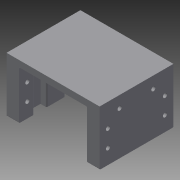
# Autodesk Inventor part: BaseMount
Saved by Autodesk Inventor 2015 (Build 190159000, 159)
## iProperties
Created: 2016-12-14
Part Number: BaseMount
Material: Generic
Document SubType Name: Modeling
Designer: Rudge-Top
Density: 1 g/cm^3
Appearance: Default
Author: Rudge-Top
Autodesk Inventor part; units mm, degrees
ref_plane "YZ Plane" through (0, 0, 0) normal (1, 0, 0) x (0, 1, 0)
ref_plane "XZ Plane" through (0, 0, 0) normal (0, 1, 0) x (-1, 0, 0)
ref_plane "XY Plane" through (0, 0, 0) normal (0, 0, 1) x (1, 0, 0)
sketch "Sketch1" plane through (0, 0, 0) normal (1, 0, 0) x (0, 1, 0)
  line L0 (0, 0) -> (-35, 0)
  line L1 (-35, 0) -> (-35, -23)
  line L2 (-35, -23) -> (0, -23)
  line L3 (0, -23) -> (0, 0)
  dimension "d0" = 35
  dimension "d1" = 23
  constraints: 8 end point, 2 parallel, 1 horizontal, 1 perpendicular
  measures "d0" distance of L2.end L1.end
  measures "d1" distance of L1.end L0.end
extrude "Extrusion1" add sketch "Sketch1" along normal blind 3
sketch "Sketch2" plane through (3, 0, 0) normal (1, 0, 0) x (0, 0, -1)
  line L0 (0, 0) -> (-3, 0)
  line L1 (-3, 0) -> (-3, -35)
  line L2 (-3, -35) -> (0, -35)
  line L3 (0, -35) -> (0, 0)
  dimension "d4" = 3
  dimension "d5" = 35
  constraints: 8 end point, 2 parallel, 1 horizontal, 1 perpendicular
  measures "d4" distance of L2.end L1.end
  measures "d5" distance of L1.end L0.end
extrude "Extrusion2" add sketch "Sketch2" against normal blind 44.1
sketch "Sketch3" plane through (0, -35, 0) normal (0, 0, -1) x (-1, 0, 0)
  line L0 (41.1, 0) -> (38.1, 0)
  line L1 (38.1, 0) -> (38.1, 35)
  line L2 (38.1, 35) -> (41.1, 35)
  line L3 (41.1, 35) -> (41.1, 0)
  point P0 (0, 35)
  dimension "d11" = 21
  dimension "d12" = 4.9
  dimension "d13" = 7
  dimension "d8" = 3
  constraints: 8 end point, 2 parallel, 1 horizontal, 1 perpendicular
  measures "d8" distance of L1.end L2.end
extrude "Extrusion3" add sketch "Sketch3" along normal blind 23
sketch "Sketch4" plane through (0, 0, 0) normal (-1, 0, 0) x (0, 0, 1)
  line L0 (0, 0) -> (0, -35) projected
  line L1 (-23, 0) -> (0, 0) projected
  line L2 (-23, -35) -> (-23, 0) projected
  line L3 (0, -35) -> (-23, -35) projected
  line L4 (0, -28) -> (-23, -28)
  line L5 (-23, -28) -> (-23, -7)
  line L6 (-23, -7) -> (0, -7)
  line L7 (0, -7) -> (0, -28)
  line L8 (-4.9, -28) -> (-4.9, -7)
  dimension "d11" = 21
  dimension "d12" = 4.9
  dimension "d13" = 7
  constraints: 10 end point, 4 point on line, 2 parallel, 2 perpendicular, 1 horizontal
  measures "d11" distance of L4.end L5.end
  measures "d12" distance between parallel lines of L0 L8
  measures "d13" distance between parallel lines of L3 L4
extrude "Extrusion4" add sketch "Sketch4" along normal blind 2.9 contours L0 L6 L2 L1 | L0 L4 L8 L6 | L0 L3 L2 L4
sketch "Sketch5" plane through (-38.1, -35, 0) normal (1, 0, 0) x (0, 0, -1)
  line L0 (0, 0) -> (0, 35) projected
  line L1 (0, 0) -> (23, 0) projected
  line L2 (23, 35) -> (23, 0) projected
  line L3 (0, 35) -> (23, 35) projected
  line L4 (0, 17.5) -> (23, 17.5)
  line L5 (5.9, 21.9028) -> (23, 21.9028)
  line L6 (23, 21.9028) -> (23, 27.9028)
  line L7 (23, 27.9028) -> (5.9, 27.9028)
  line L8 (5.9, 27.9028) -> (5.9, 21.9028)
  line L9 (23, 0) -> (23, 35)
  line L10 (5.9, 13.0972) -> (23, 13.0972)
  line L11 (23, 7.0972) -> (5.9, 7.0972)
  line L12 (5.9, 7.0972) -> (5.9, 13.0972)
  line L13 (23, 13.0972) -> (23, 7.0972)
  line L14 (23, 35) -> (23, 0) projected
  dimension "d16" = 6
  dimension "d17" = 0
  dimension "d18" = 5.9
  constraints: 20 end point, 6 symmetric about line, 2 midpoint, 2 parallel, 1 collinear, 1 horizontal, 1 perpendicular
  measures "d16" distance of L6.end L5.end
  measures "d17" distance between parallel lines of L2 L6
  measures "d18" distance between parallel lines of L0 L8
extrude "Extrusion5" add sketch "Sketch5" along normal blind 2.9 contours L0 L4 L2 L10 L12 L11 L1 | L0 L3 L2 L7 L8 L5 L4
fillet "Fillet1" radius 0.5 2 edges at (-2.9, -17.5, 0) (-35.2, -17.5, 0)
fillet "Fillet2" radius 0.5 6 edges at (-1.45, -7, -4.9) (-1.45, -28, -4.9) (-36.65, -7.0972, -5.9) (-36.65, -13.0972, -5.9) (-36.65, -21.9028, -5.9) (-35.2, -27.9028, -14.45)
sketch "Sketch6" plane through (3, 0, 0) normal (1, 0, 0) x (0, 0, -1)
  line L0 (-3, -35) -> (23, -35) projected
  line L1 (23, -35) -> (23, 0) projected
  line L2 (23, 0) -> (-3, 0) projected
  line L3 (-3, 0) -> (-3, -35) projected
  line L4 (23, -28) -> (23, -7) projected
  line L5 (23, -17.5) -> (9.3491, -17.5)
  line L6 (5.9, -28.4028) -> (23, -28.4028) projected
  line L7 (5.9, -28.4028) -> (5.9, -22.4028) projected
  arc A0 (6.4, -21.9028) -> (5.9, -22.4028) centre (6.4, -22.4028) ccw projected
  line L8 (6.4, -21.9028) -> (23, -21.9028) projected
  line L9 (23, -21.9028) -> (23, -13.0972) projected
  line L10 (23, -13.0972) -> (6.4, -13.0972) projected
  arc A1 (5.9, -12.5972) -> (6.4, -13.0972) centre (6.4, -12.5972) ccw projected
  line L11 (5.9, -12.5972) -> (5.9, -7.5972) projected
  arc A2 (6.4, -7.0972) -> (5.9, -7.5972) centre (6.4, -7.5972) ccw projected
  line L12 (6.4, -7.0972) -> (23, -7.0972) projected
  line L13 (23, -7.0972) -> (23, 0) projected
  line L14 (23, 0) -> (0.5, 0) projected
  line L15 (0.5, -35) -> (0.5, 0) projected
  line L16 (0.5, -35) -> (23, -35) projected
  line L17 (23, -35) -> (23, -28.4028) projected
  line L18 (0, -35) -> (0.5, -35) projected
  line L19 (0.5, -35) -> (0.5, 0) projected
  line L20 (0.5, 0) -> (0, 0) projected
  line L21 (0, 0) -> (0, -35) projected
  point P0 (2.5, -25.5)
  point P1 (16, -31)
  point P2 (8, -31)
  point P3 (2.5, -9.5)
  point P4 (16, -4)
  point P5 (8, -4)
  dimension "d23" = 8
  dimension "d24" = 2.5
  dimension "d25" = 5.5
  dimension "d26" = 8
  dimension "d27" = 13.5
  dimension "d28" = 13.5
  constraints: 3 symmetric about line, 2 end point, 1 horizontal, 1 midpoint
  measures "d23" distance from line of point (2.5, -25.5) L5
  measures "d24" distance from line of point (2.5, -25.5) L21
  measures "d25" horizontal distance of point (2.5, -25.5) point (8, -31)
  measures "d26" distance of point (16, -31) point (8, -31)
  measures "d27" distance from line of L5 point (8, -31)
  measures "d28" distance from line of L5 point (16, -31)
hole "Hole1" at (3, -25.5, -2.5) at (3, -31, -16) at (3, -31, -8) at (3, -4, -16) at (3, -4, -8) at (3, -9.5, -2.5) direction (-1, 0, 0) diameter 2 end through all
fillet "Fillet3" radius 0.5 27 edges at (-38.15, 0, -23) (-36.65, -7.0972, -23) (-36.65, -13.0972, -23) (-35.2, -22.0492, -6.0464) (-35.2, -25.4028, -5.9) (-35.2, -21.9028, -14.7) (-35.2, -12.9508, -6.0464) (-35.2, -10.0972, -5.9) (-35.2, -7.2437, -6.0464) (-35.2, -7.0972, -14.7) (-35.2, -13.0972, -14.7) (-38.15, -35, -23) (0.05, 0, -23) (-1.45, -7, -23) (0, -17.5, -23) (-1.45, -28, -23) (0, -7.1464, -5.0464) (0, -7, -14.2) (0, -27.8536, -5.0464) (0, -28, -14.2) (0, -17.5, -4.9) (-2.9, -27.8536, -5.0464) (-2.9, -28, -14.2) (-2.9, -7.1464, -5.0464) (-2.9, -7, -14.2) (-2.9, -17.5, -4.9) (0.05, -35, -23)
body "Solid1"
